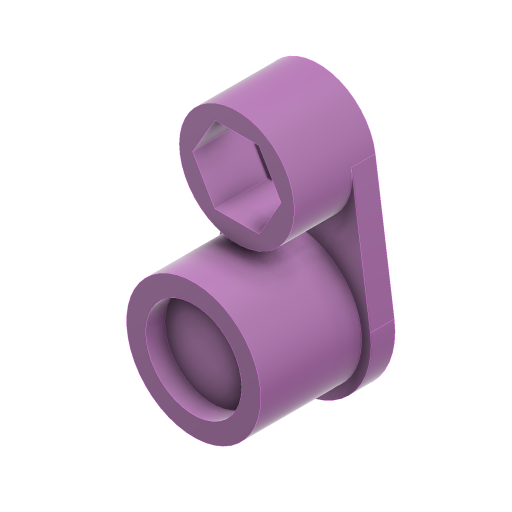
# Autodesk Inventor part: Капсула
Saved by Autodesk Inventor 2024.1 (Build 281209000, 209)
## iProperties
Created: 2023-06-09
Part Number: Капсула
Material: Типовые
Document SubType Name: Modeling
Designer: Admin
Density: 1 g/cm^3
Appearance: По умолчанию
External_diam: 16,000 мм
External_nut_holder: 12,000 мм
Hole: 5,000 мм
Legnth: 14,219 мм
Nut: 8,000 мм
Depth: 6,000 мм
Nut_thick: 0,500 мм
Magnet_fit: 10,000 мм
External_mag_holder: 14,000 мм
Author: Admin
Autodesk Inventor part; units mm, degrees
ref_plane "YZ Plane" through (0, 0, 0) normal (1, 0, 0) x (0, 1, 0)
ref_plane "XZ Plane" through (0, 0, 0) normal (0, 1, 0) x (-1, 0, 0)
ref_plane "XY Plane" through (0, 0, 0) normal (0, 0, 1) x (1, 0, 0)
sketch "Эскиз1" plane through (0, 0, 0) normal (0, 0, 1) x (1, 0, 0)
  arc A0 (-7.9205, 1.1252) -> (7.9205, 1.1252) centre (0, 0) ccw
  circle A1 centre (0, 14.2191) radius 6
  line L0 (7.9205, 1.1252) -> (5.9404, 15.0631)
  line L1 (-7.9205, 1.1252) -> (-5.9404, 15.0631)
  circle A2 centre (0, 0) radius 7
  arc A3 (7.9205, 1.1252) -> (-7.9205, 1.1252) centre (0, 0) ccw construction
  circle A4 centre (0, 14.2191) radius 2.5
  line L2 (2.3094, 18.2191) -> (4.6188, 14.2191)
  line L3 (4.6188, 14.2191) -> (2.3094, 10.2191)
  line L4 (2.3094, 10.2191) -> (-2.3094, 10.2191)
  line L5 (-2.3094, 10.2191) -> (-4.6188, 14.2191)
  line L6 (-4.6188, 14.2191) -> (-2.3094, 18.2191)
  line L7 (-2.3094, 18.2191) -> (2.3094, 18.2191)
  circle A5 centre (0, 0) radius 5
  point P0 (-5.6643, 4.1129)
  point P1 (-6.8918, 1.226)
  point P2 (-6.9958, -0.2431)
  point P3 (-5.2611, 17.1038)
  point P4 (-5.7507, 15.9307)
  point P5 (-5.9065, 15.2742)
  constraints: 16 end point, 14 point on circle, 6 centre point, 5 coincident, 4 tangent, 2 vertical alignment, 1 horizontal, 1 parallel, 18 other
extrude "Выдавливание1" add sketch "Эскиз1" against normal blind 2.5 contours L1 A1 L0 A0 | A1 | A2 | A4 | L2 L3 L4 L5 L6 L7 | A5
extrude "Выдавливание2" cut sketch "Эскиз1" against normal blind 1 contours A4
extrude "Выдавливание3" add sketch "Эскиз1" along normal blind 6 contours A1
extrude "Выдавливание4" add sketch "Эскиз1" along normal blind 0.5 contours L2 L3 L4 L5 L6 L7
extrude "Выдавливание5" add sketch "Эскиз1" along normal blind 10.5 contours A2
extrude "Выдавливание7" add sketch "Эскиз1" along normal blind 8.5 contours A5
